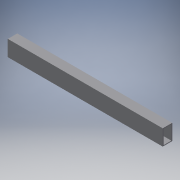
# Autodesk Inventor part: suport for a piston
Saved by Autodesk Inventor 2017 (Build 210142000, 142)
## iProperties
Created: 2019-02-05
Part Number: suport for a piston
Material: Generic
Document SubType Name: Modeling
Designer: S346852600
Density: 1 g/cm^3
Appearance: Default
Author: S346852600
Autodesk Inventor part; units mm, degrees
ref_plane "YZ Plane" through (0, 0, 0) normal (1, 0, 0) x (0, 1, 0)
ref_plane "XZ Plane" through (0, 0, 0) normal (0, 1, 0) x (-1, 0, 0)
ref_plane "XY Plane" through (0, 0, 0) normal (0, 0, 1) x (1, 0, 0)
sketch "Sketch1" plane through (0, 0, 0) normal (1, 0, 0) x (0, 1, 0)
  line L0 (0, 0) -> (-63.5, 0)
  line L1 (-63.5, 0) -> (-63.5, -38.1)
  line L2 (-63.5, -38.1) -> (0, -38.1)
  line L3 (0, -38.1) -> (0, 0)
  line L4 (-3.175, -3.175) -> (-60.325, -3.175)
  line L5 (-60.325, -3.175) -> (-60.325, -34.925)
  line L6 (-60.325, -34.925) -> (-3.175, -34.925)
  line L7 (-3.175, -34.925) -> (-3.175, -3.175)
  dimension "d0" = 63.5
  dimension "d1" = 38.1
  dimension "d2" = 3.175
  constraints: 16 end point, 4 parallel, 2 perpendicular, 1 horizontal, 3 other
  measures "d0" distance of L2.end L1.end
  measures "d1" distance of L1.end L0.end
  measures "d2" distance between parallel lines of L3 L7
extrude "Extrusion1" add sketch "Sketch1" along normal blind 622.3
body "Solid1"
